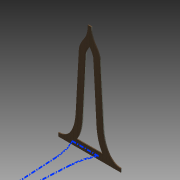
# Autodesk Inventor part: Top Plate
Saved by Autodesk Inventor 2013 SP1 (Build 170176100, 176)
## iProperties
Created: 2013-02-28
Part Number: Top Plate
Material: Wood (Cherry)
Document SubType Name: Modeling
Designer: fixer
Mass: 47.8412 g
Surface Area: 653.113 cm^2
Volume: 95.6825 cm^3
Density: 0.5 g/cm^3
Author: fixer
Autodesk Inventor part; units mm, degrees
ref_plane "YZ Plane" through (0, 0, 0) normal (1, 0, 0) x (0, 1, 0)
ref_plane "XZ Plane" through (0, 0, 0) normal (0, 1, 0) x (-1, 0, 0)
ref_plane "XY Plane" through (0, 0, 0) normal (0, 0, 1) x (1, 0, 0)
derived "Bottom Plate v2.ipt"
sketch "Sketch1_1" plane through (0, 0, 0) normal (0, 0, 1) x (1, 0, 0)
  line L0 (76.2, -12.7) -> (381, -12.7) construction
  line L1 (-76.2, -12.7) -> (-381, -12.7) construction
  line L2 (-76.2, 0) -> (-381, 0) construction
  line L3 (76.2, 0) -> (381, 0) construction
  line L4 (0, -116.2267) -> (0, 608.4603) construction
  line L5 (0, -12.7) -> (-114.3, -12.7)
  line L6 (-114.3, -12.7) -> (-114.3, 0)
  line L7 (0, 406.4) -> (-6.35, 406.4)
  line L8 (-39.0138, 312.42) -> (-50.5988, 93.6374)
  line L9 (39.0138, 312.42) -> (50.5988, 93.6374)
  line L10 (0, 406.4) -> (6.35, 406.4)
  line L11 (0, -12.7) -> (114.3, -12.7)
  line L12 (114.3, -12.7) -> (114.3, 0)
  spline S0 degree 4 poles (-6.35, 406.4) (-6.35, 374.2572) (-17.7644, 366.5849) (-7.7511, 356.5096) (-38.295, 325.9934) (-39.0138, 312.42) knots 0 0 0 0 0 0.493995 1 1 1 1 1
  spline S1 degree 4 poles (6.35, 406.4) (6.35, 374.2572) (17.7644, 366.5849) (7.7511, 356.5096) (38.295, 325.9934) (39.0138, 312.42) knots 0 0 0 0 0 0.493995 1 1 1 1 1
  spline S2 degree 3 poles (-50.5988, 93.6374) (-52.7393, 53.2143) (-67.314, 0) (-114.3, 0) knots 0 0 0 0 1 1 1 1
  spline S3 degree 3 poles (50.5988, 93.6374) (52.7393, 53.2143) (67.314, 0) (114.3, 0) knots 0 0 0 0 1 1 1 1
  line L13 (19.05, 12.7) -> (-19.05, 12.7)
  line L14 (-19.05, 12.7) -> (-19.05, 23.9218)
  line L15 (-19.05, 23.9218) -> (19.05, 23.9218)
  line L16 (19.05, 23.9218) -> (19.05, 12.7)
  line L17 (-19.05, 20.9628) -> (19.05, 20.9628) construction
  line L18 (-12.7, 158.2448) -> (-12.7, 218.4428) construction
  line L19 (12.7, 158.2448) -> (-12.7, 158.2448) construction
  line L20 (12.7, 218.4428) -> (12.7, 158.2448) construction
  line L21 (-12.7, 218.4428) -> (12.7, 218.4428) construction
  line L22 (-38.1, 12.7) -> (38.1, 12.7) construction
  line L23 (0, 96.1517) -> (23.388, 96.1517)
  line L24 (28.4609, 101.5003) -> (22.0411, 222.7364)
  line L25 (16.9683, 227.5478) -> (0, 227.5478)
  line L26 (0, 96.1517) -> (-23.388, 96.1517)
  line L27 (-28.4609, 101.5003) -> (-22.0411, 222.7364)
  line L28 (-16.9683, 227.5478) -> (0, 227.5478)
  arc A0 (-16.9683, 227.5478) -> (-22.0411, 222.7364) centre (-16.9683, 222.4678) ccw
  arc A1 (22.0411, 222.7364) -> (16.9683, 227.5478) centre (16.9683, 222.4678) ccw
  arc A2 (23.388, 96.1517) -> (28.4609, 101.5003) centre (23.388, 101.2317) ccw
  arc A3 (-28.4609, 101.5003) -> (-23.388, 96.1517) centre (-23.388, 101.2317) ccw
  point P0 (0, 0)
  point P1 (-14.9241, 359.2979)
  point P2 (14.9241, 359.2979)
  point P3 (0, 12.7)
  point P4 (28.7441, 96.1517)
  point P5 (21.7864, 227.5478)
  point P6 (-28.7441, 96.1517)
  point P7 (-21.7864, 227.5478)
  dimension "d9" = 5.08
  measures "d9" radius of A0
extrude "Extrusion2" add sketch "Sketch1_1" along normal blind 3.175
body "Solid1"
